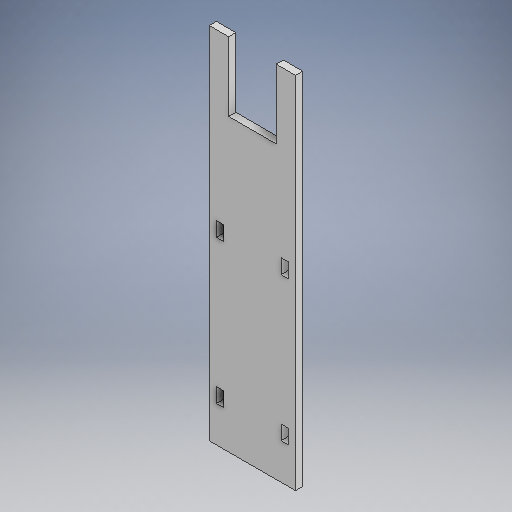
# Autodesk Inventor part: Lifting Sections left
Saved by Autodesk Inventor 2025.3 (Build 293356000, 356)
## iProperties
Created: 2026-04-06
Part Number: Lifting Sections left
Material: Generic
Document SubType Name: Modeling
Designer: user
Density: 1 g/cm^3
Appearance: Default
Author: user
Autodesk Inventor part; units mm, degrees
ref_plane "YZ Plane" through (0, 0, 0) normal (1, 0, 0) x (0, 1, 0)
ref_plane "XZ Plane" through (0, 0, 0) normal (0, 1, 0) x (-1, 0, 0)
ref_plane "XY Plane" through (0, 0, 0) normal (0, 0, 1) x (1, 0, 0)
sketch "Sketch1" plane through (0, 0, 0) normal (0, 0, 1) x (1, 0, 0)
  line L0 (-61.8733, -121.208) -> (-61.8733, 128.792)
  line L1 (-61.8733, 128.792) -> (-1.8733, 128.792)
  line L2 (-1.8733, 128.792) -> (-1.8733, -121.208)
  line L3 (-1.8733, -121.208) -> (-61.8733, -121.208)
  line L4 (-66.8733, 113.892) -> (-51.7733, 113.892) construction
  line L5 (-66.8733, 103.792) -> (-1.8733, 103.792) construction
  line L6 (-56.8733, -86.108) -> (-51.7733, -86.108)
  line L7 (-51.7733, -96.208) -> (-56.8733, -96.208)
  line L8 (-51.7733, 13.892) -> (-56.8733, 13.892)
  line L9 (-51.7733, 3.792) -> (-56.8733, 3.792)
  line L10 (-51.7733, 3.792) -> (-51.7733, -86.108) construction
  line L11 (-56.8733, 3.792) -> (-56.8733, -86.108) construction
  line L12 (-51.7733, 13.892) -> (-51.7733, 3.792)
  line L13 (-56.8733, 13.892) -> (-56.8733, 3.792)
  line L14 (-51.7733, 103.792) -> (-51.7733, 13.892) construction
  line L15 (-56.8733, 103.792) -> (-56.8733, 80.792) construction
  line L16 (-51.7733, -86.108) -> (-51.7733, -96.208)
  line L17 (-56.8733, -86.108) -> (-56.8733, -96.208)
  line L18 (-31.8733, 128.792) -> (-31.8733, -121.208) construction
  line L19 (3.1267, 103.792) -> (-61.8733, 103.792) construction
  line L20 (3.1267, 113.892) -> (-61.8733, 113.892) construction
  line L21 (-11.9733, 13.892) -> (-6.8733, 13.892)
  line L22 (-11.9733, 3.792) -> (-6.8733, 3.792)
  line L23 (-11.9733, 13.892) -> (-11.9733, 3.792)
  line L24 (-6.8733, 13.892) -> (-6.8733, 3.792)
  line L25 (-6.8733, -86.108) -> (-6.8733, -96.208)
  line L26 (-6.8733, -86.108) -> (-11.9733, -86.108)
  line L27 (-11.9733, -86.108) -> (-11.9733, -96.208)
  line L28 (-11.9733, -96.208) -> (-6.8733, -96.208)
  line L29 (-1.8733, 128.792) -> (-6.8733, 128.792)
  line L30 (-51.7733, 113.892) -> (-1.8733, 113.892) construction
  line L31 (-61.8733, 128.792) -> (-56.8733, 128.792)
  line L32 (-31.8733, 80.792) -> (-48.3733, 80.792)
  line L33 (-48.3733, 80.792) -> (-48.3733, 128.792)
  line L34 (-31.8733, 80.792) -> (-15.3733, 80.792)
  line L35 (-15.3733, 80.792) -> (-15.3733, 128.792)
  point P0 (0, 0)
  point P1 (-56.8733, 92.292)
  dimension "d6" = 60
  dimension "d7" = 5
  dimension "d11" = 48
  dimension "d12" = 39.8
  dimension "d16" = 25
  dimension "d17" = 16.5
  dimension "d18" = 16.5
  constraints: 72 end point, 12 symmetric about line, 8 point on line, 6 perpendicular, 5 vertical, 4 horizontal, 3 midpoint, 1 collinear, 1 parallel
  measures "d6" distance of L0.end L2.start
  measures "d7" distance between parallel lines of L0 L13
  measures "d11" distance of L31.end L15.end
  measures "d12" distance between parallel lines of L23 L12
  measures "d16" distance from line of L18 point (-56.873, 92.292)
  measures "d17" distance of L32.start L32.end
  measures "d18" distance of L32.start L34.end
extrude "Extrusion1" add sketch "Sketch1" along normal blind 5 contours L0 L1 L33 L32 L34 L35 L2 L3
body "Solid1"
